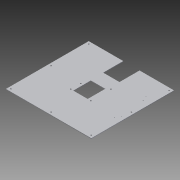
# Autodesk Inventor part: New BottomHopper Plate
Saved by Autodesk Inventor 2013 (Build 170138000, 138)
## iProperties
Created: 2013-07-19
Part Number: New BottomHopper Plate
Material: Aluminum 6061
Document SubType Name: Modeling
Designer: nowireless
Density: 1 g/cm^3
Author: nowireless
Autodesk Inventor part; units mm, degrees
ref_plane "YZ Plane" through (0, 0, 0) normal (1, 0, 0) x (0, 1, 0)
ref_plane "XZ Plane" through (0, 0, 0) normal (0, 1, 0) x (-1, 0, 0)
ref_plane "XY Plane" through (0, 0, 0) normal (0, 0, 1) x (1, 0, 0)
sketch "Sketch1" plane through (0, 0, 0) normal (0, 1, 0) x (-1, 0, 0)
  line L0 (0, 0) -> (431.8, 0)
  line L1 (431.8, 0) -> (431.8, 431.8)
  line L2 (431.8, 431.8) -> (0, 431.8)
  line L3 (0, 431.8) -> (0, 0)
  dimension "d0" = 431.8
  dimension "d2" = 431.8
  constraints: 8 end point, 2 parallel, 1 horizontal, 1 perpendicular
  measures "d0" distance of L1.end L2.end
  measures "d2" distance of L2.end L0.start
extrude "Extrusion1" add sketch "Sketch1" along normal blind 3.175
sketch "Sketch2" plane through (0, 3.175, 0) normal (0, 1, 0) x (1, 0, 0)
  line L0 (0, 0) -> (-431.8, 0) projected
  line L1 (-431.8, 0) -> (-431.8, -431.8) projected
  line L2 (-431.8, -431.8) -> (0, -431.8) projected
  line L3 (0, -431.8) -> (0, 0) projected
  line L4 (-257.175, -114.3) -> (-174.625, -114.3)
  line L5 (-174.625, -114.3) -> (-174.625, -19.05)
  line L6 (-257.175, -31.75) -> (-257.175, -114.3)
  line L7 (0, -215.9) -> (-431.8, -215.9)
  line L8 (-174.625, 0) -> (-174.625, -19.05)
  line L9 (-257.175, -31.75) -> (-257.175, 0)
  line L10 (-215.9, -431.8) -> (-215.9, -215.9)
  dimension "d5" = 82.55
  dimension "d7" = 82.55
  dimension "d8" = 215.9
  dimension "d9" = 101.6
  dimension "d10" = 41.275
  dimension "d51" = 174.625
  dimension "d52" = 174.625
  constraints: 14 end point, 4 midpoint, 4 perpendicular, 2 point on line, 1 horizontal, 1 parallel
  measures "d5" distance of L6.start L4.start
  measures "d7" distance of L4.start L4.end
  measures "d8" distance between parallel lines of L7 L0
  measures "d9" distance between parallel lines of L7 L4
  measures "d10" distance between parallel lines of L5 L10
  measures "d51" distance between parallel lines of L3 L5
  measures "d52" distance between parallel lines of L1 L6
extrude "Extrusion2" cut sketch "Sketch2" against normal blind 3.175 contours L8 L5 L4 L6 L9 L0
sketch "Sketch3" plane through (0, 3.175, 0) normal (0, 1, 0) x (1, 0, 0)
  line L0 (-431.8, 0) -> (-431.8, -431.8) projected
  line L1 (-431.8, -431.8) -> (0, -431.8) projected
  line L2 (-266.7, -268.7828) -> (-165.1, -268.7828)
  line L3 (-165.1, -268.7828) -> (-165.1, -167.1828)
  line L4 (-165.1, -167.1828) -> (-266.7, -167.1828)
  line L5 (-266.7, -167.1828) -> (-266.7, -268.7828)
  line L6 (-215.9, -167.1828) -> (-215.9, -268.7828)
  line L7 (-165.1, -217.9828) -> (-266.7, -217.9828)
  line L8 (0, -431.8) -> (0, 0) projected
  dimension "d13" = 101.6
  dimension "d15" = 101.6
  dimension "d18" = 215.9
  dimension "d19" = 213.8172
  dimension "d55" = 50.8
  dimension "d56" = 50.8
  dimension "d57" = 215.9
  constraints: 12 end point, 4 coincident, 4 midpoint, 2 parallel, 1 horizontal, 1 perpendicular
  measures "d13" distance of L2.start L2.end
  measures "d15" distance of L2.end L3.end
  measures "d18" distance between parallel lines of L0 L6
  measures "d19" distance between parallel lines of L1 L7
  measures "d55" distance between parallel lines of L2 L7
  measures "d56" distance between parallel lines of L5 L6
  measures "d57" distance between parallel lines of L8 L6
hole "Hole1" at (-165.1, 3.175, 167.1828) at (-266.7, 3.175, 217.9828) at (-266.7, 3.175, 268.7828) at (-165.1, 3.175, 268.7828) direction (0, -1, 0) diameter 6.35 end through all
sketch "Sketch4" plane through (0, 3.175, 0) normal (0, 1, 0) x (1, 0, 0)
  circle A0 centre (-165.1, -167.1828) radius 3.175 projected
  circle A1 centre (-266.7, -217.9828) radius 3.175 projected
  circle A2 centre (-165.1, -268.7828) radius 3.175 projected
  line L0 (-254, -268.7828) -> (-180.975, -268.7828)
  line L1 (-180.975, -268.7828) -> (-180.975, -179.8828)
  line L2 (-180.975, -179.8828) -> (-254, -179.8828)
  line L3 (-254, -179.8828) -> (-254, -268.7828)
  line L4 (-431.8, 0) -> (-431.8, -431.8) projected
  line L5 (0, -431.8) -> (0, 0) projected
  dimension "d27" = 12.7
  dimension "d28" = 12.7
  dimension "d29" = 12.7
  dimension "d30" = 88.9
  dimension "d53" = 177.8
  dimension "d54" = 180.975
  constraints: 8 end point, 2 parallel, 1 horizontal, 1 perpendicular
  measures "d27" distance from line of A1.centre L3
  measures "d28" distance edge to line of A2 L1
  measures "d29" distance from line of L2 A0.centre
  measures "d30" distance of L0.end L1.end
  measures "d53" distance between parallel lines of L4 L3
  measures "d54" distance between parallel lines of L5 L1
extrude "Extrusion3" cut sketch "Sketch4" against normal blind 3.175 contours L3 L2 L1 L0
sketch "Sketch5" plane through (0, 3.175, 0) normal (0, 1, 0) x (1, 0, 0)
  line L0 (-431.8, 0) -> (-431.8, -431.8) projected
  line L1 (-431.8, -431.8) -> (0, -431.8) projected
  line L2 (0, -431.8) -> (0, 0) projected
  point P0 (-419.1, -215.9)
  point P1 (-215.9, -419.1)
  point P2 (-12.7, -215.9)
  dimension "d33" = 12.7
  dimension "d34" = 12.7
  dimension "d35" = 12.7
  dimension "d36" = 215.9
  dimension "d37" = 215.9
  dimension "d38" = 215.9
  measures "d33" distance from line of L0 point (-419.1, -215.9)
  measures "d34" distance from line of L1 point (-215.9, -419.1)
  measures "d35" distance from line of point (-12.7, -215.9) L2
  measures "d36" distance from line of point (-419.1, -215.9) L1
  measures "d37" distance from line of L1 point (-12.7, -215.9)
  measures "d38" distance from line of point (-215.9, -419.1) L2
hole "Hole2" at (-419.1, 3.175, 215.9) at (-215.9, 3.175, 419.1) at (-12.7, 3.175, 215.9) direction (0, -1, 0) diameter 6.35 end through all
sketch "Sketch6" plane through (0, 3.175, 0) normal (0, 1, 0) x (1, 0, 0)
  line L0 (0, -431.8) -> (0, 0) projected
  line L1 (0, 0) -> (-174.625, 0) projected
  line L2 (-174.625, 0) -> (-174.625, -114.3) projected
  line L3 (-174.625, -12.7) -> (0, -12.7)
  dimension "d46" = 12.7
  constraints: 2 end point, 2 point on line, 1 perpendicular
  measures "d46" distance between parallel lines of L3 L1
extrude "Extrusion4" cut sketch "Sketch6" against normal blind 25.4
sketch "Sketch7" plane through (0, 3.175, 0) normal (0, 1, 0) x (1, 0, 0)
  line L0 (-257.175, -114.3) -> (-257.175, 0) projected
  line L1 (-257.175, 0) -> (-431.8, 0) projected
  line L2 (-431.8, 0) -> (-431.8, -431.8) projected
  line L3 (-257.175, -12.7) -> (-431.8, -12.7)
  point P0 (0, 0)
  dimension "d58" = 12.7
  constraints: 2 end point, 2 point on line, 1 perpendicular
  measures "d58" distance between parallel lines of L3 L1
extrude "Extrusion5" cut sketch "Sketch7" against normal blind 25.4
sketch "Sketch8" plane through (0, 3.175, 0) normal (0, 1, 0) x (1, 0, 0)
  line L0 (-257.175, -12.7) -> (-431.8, -12.7) projected
  line L1 (-431.8, -12.7) -> (-431.8, -431.8) projected
  line L2 (-431.8, -431.8) -> (0, -431.8) projected
  line L3 (0, -431.8) -> (0, -12.7) projected
  line L4 (0, -12.7) -> (-174.625, -12.7) projected
  point P0 (0, 0)
  point P1 (-419.1, -25.4)
  point P2 (-12.7, -25.4)
  point P3 (-419.1, -419.1)
  point P4 (-12.7, -419.1)
  dimension "d59" = 12.7
  dimension "d60" = 12.7
  dimension "d61" = 12.7
  dimension "d62" = 12.7
  dimension "d63" = 12.7
  dimension "d64" = 12.7
  dimension "d65" = 12.7
  dimension "d66" = 12.7
  measures "d59" distance from line of point (-419.1, -25.4) L1
  measures "d60" distance from line of L0 point (-419.1, -25.4)
  measures "d61" distance from line of L4 point (-12.7, -25.4)
  measures "d62" distance from line of point (-12.7, -25.4) L3
  measures "d63" distance from line of point (-419.1, -419.1) L1
  measures "d64" distance from line of L2 point (-419.1, -419.1)
  measures "d65" distance from line of L2 point (-12.7, -419.1)
  measures "d66" distance from line of L3 point (-12.7, -419.1)
hole "Hole3" at (-419.1, 3.175, 25.4) at (-12.7, 3.175, 25.4) at (-419.1, 3.175, 419.1) at (-12.7, 3.175, 419.1) direction (0, -1, 0) diameter 6.35 end through all
sketch "Sketch9" plane through (0, 0, 0) normal (0, -1, 0) x (1, 0, 0)
  line L0 (0, 431.8) -> (0, 12.7) projected
  point P0 (0, 0)
  point P1 (-34.29, 134.8443)
  dimension "d74" = 34.29
  measures "d74" distance from line of L0 point (-34.29, 134.844)
hole "Hole4" at (-34.29, 0, 134.8443) direction (0, 1, 0) diameter 3 end through all
sketch "Sketch10" plane through (0, 0, 0) normal (0, -1, 0) x (1, 0, 0)
  line L0 (0, 431.8) -> (0, 12.7) projected
  point P0 (0, 0)
  point P1 (-31.75, 281.1231)
  dimension "d82" = 31.75
  measures "d82" distance from line of L0 point (-31.75, 281.123)
hole "Hole5" at (-31.75, 0, 281.1231) direction (0, 1, 0) diameter 3 end through all
sketch "Sketch12" plane through (0, 0, 0) normal (0, -1, 0) x (1, 0, 0)
  circle A0 centre (-34.29, 134.8443) radius 1.5 projected
  line L0 (0, 431.8) -> (0, 12.7) projected
  line L1 (-34.29, 134.8443) -> (-50.0054, 119.1289)
  line L2 (-50.0054, 119.1289) -> (-42.7314, 111.8548)
  point P0 (0, 0)
  dimension "d108" = 45
  dimension "d109" = 22.225
  dimension "d110" = 10.287
  constraints: 4 end point, 1 coincident, 1 perpendicular
  measures "d108" angle of L0 L1
  measures "d109" distance of L1.start L1.end
  measures "d110" distance of L1.end L2.end
hole "Hole7" at (-42.7314, 0, 111.8548) direction (0, 1, 0) diameter 3 depth 25.4 tip angle 118
sketch "Sketch13" plane through (0, 0, 0) normal (0, -1, 0) x (1, 0, 0)
  circle A0 centre (-31.75, 281.1231) radius 1.5 projected
  line L0 (0, 431.8) -> (0, 12.7) projected
  line L1 (-31.75, 281.1231) -> (-30.1997, 258.9522)
  line L2 (-30.1997, 258.9522) -> (-19.9377, 259.6698)
  point P0 (0, 0)
  dimension "d118" = 4
  dimension "d119" = 22.225
  dimension "d120" = 10.287
  constraints: 4 end point, 1 coincident, 1 perpendicular
  measures "d118" angle of L0 L1
  measures "d119" distance of L1.start L1.end
  measures "d120" distance of L1.end L2.end
hole "Hole8" at (-19.9377, 0, 259.6698) direction (0, 1, 0) diameter 3 depth 25.4 tip angle 118
body "Solid1"
